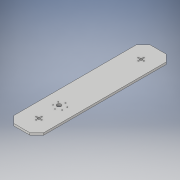
# Autodesk Inventor part: testPart_chassis2
Saved by Autodesk Inventor 2019 (Build 230136000, 136)
## iProperties
Created: 2019-09-17
Part Number: testPart_chassis2
Material: Generic
Document SubType Name: Modeling
Designer: shrey
Density: 1 g/cm^3
Appearance: Default
Author: shrey
Autodesk Inventor part; units mm, degrees
ref_plane "YZ Plane" through (0, 0, 0) normal (1, 0, 0) x (0, 1, 0)
ref_plane "XZ Plane" through (0, 0, 0) normal (0, 1, 0) x (-1, 0, 0)
ref_plane "XY Plane" through (0, 0, 0) normal (0, 0, 1) x (1, 0, 0)
sketch "Sketch1" plane through (0, 0, 0) normal (0, 1, 0) x (-1, 0, 0)
  line L0 (-44.45, -203.2) -> (44.45, -203.2)
  line L1 (44.45, -203.2) -> (44.45, 203.2)
  line L2 (44.45, 203.2) -> (-44.45, 203.2)
  line L3 (-44.45, 203.2) -> (-44.45, -203.2)
  line L4 (-44.45, -203.2) -> (44.45, 203.2) construction
  line L5 (44.45, -203.2) -> (-44.45, 203.2) construction
  line L6 (0, 203.2) -> (0, -203.2) construction
  line L7 (0, 0) -> (44.45, 0) construction
  line L8 (0, -203.2) -> (0, 203.2) construction
  line L9 (0, 152.4) -> (7.112, 152.4) construction
  line L10 (0, -152.4) -> (0, -203.2) construction
  circle A0 centre (0, -152.4) radius 4
  circle A1 centre (0, -152.4) radius 8 construction
  line L11 (0, 152.4) -> (-44.45, 152.4) construction
  line L12 (-44.45, 152.4) -> (-44.45, 88.9)
  line L13 (-44.45, 88.9) -> (0, 88.9) construction
  line L14 (0, 88.9) -> (0, 152.4) construction
  circle A2 centre (0, 88.9) radius 3.556 construction
  circle A3 centre (3.556, 88.9) radius 5.9944
  circle A4 centre (0, 88.9) radius 15.494 construction
  circle A5 centre (0, 104.394) radius 1.5
  circle A6 centre (0, 88.9) radius 15.494 construction
  circle A7 centre (-13.4182, 96.647) radius 1.5
  circle A8 centre (0, 88.9) radius 15.494 construction
  circle A9 centre (-13.4182, 81.153) radius 1.5
  circle A10 centre (0, 88.9) radius 15.494 construction
  circle A11 centre (0, 73.406) radius 1.5
  circle A12 centre (0, 88.9) radius 15.494 construction
  circle A13 centre (13.4182, 81.153) radius 1.5
  circle A14 centre (0, 88.9) radius 15.494 construction
  circle A15 centre (13.4182, 96.647) radius 1.5
  circle A16 centre (0, -144.4) radius 1.85
  circle A17 centre (-8, -152.4) radius 1.85
  circle A18 centre (0, -160.4) radius 1.85
  circle A19 centre (8, -152.4) radius 1.85
  circle A20 centre (0, 152.4) radius 4
  circle A21 centre (0, 152.4) radius 8 construction
  circle A22 centre (0, 160.4) radius 1.85
  circle A23 centre (0, 152.4) radius 8 construction
  circle A24 centre (-8, 152.4) radius 1.85
  circle A25 centre (0, 152.4) radius 8 construction
  circle A26 centre (0, 144.4) radius 1.85
  circle A27 centre (0, 152.4) radius 8 construction
  circle A28 centre (8, 152.4) radius 1.85
  dimension "d17" = 16
  dimension "d26" = 7.112
  dimension "d28" = 30.988
  dimension "d40" = 16
  dimension "d0" = 406.4
  dimension "d1" = 88.9
  dimension "d2" = 152.4
  dimension "d16" = 8
  dimension "d24" = 44.45
  dimension "d25" = 63.5
  dimension "d27" = 11.9888
  dimension "d29" = 3
  dimension "d32" = 360
  dimension "d34" = 3.7
  dimension "d37" = 360
  dimension "d39" = 8
  dimension "d41" = 3.7
  dimension "d44" = 360
  constraints: 30 end point, 17 centre point, 9 coincident, 5 midpoint, 5 vertical alignment, 4 parallel, 4 point on line, 3 horizontal, 3 horizontal alignment, 3 symmetric about line, 2 perpendicular, 1 collinear, 77 other
  measures "d0" distance of L0.end L1.end
  measures "d1" distance of L1.end L2.end
  measures "d2" distance of L7.start point (0, 152.4)
  measures "d16" diameter of A0
  measures "d24" distance of L9.start L11.end
  measures "d25" distance of L11.end L12.end
  measures "d27" diameter of A3
  measures "d29" diameter of A5
  measures "d34" diameter of A16
  measures "d39" diameter of A20
  measures "d41" diameter of A22
extrude "Extrusion2" add sketch "Sketch1" along normal blind 6.35
chamfer "Chamfer2" distance 20.32 angle 45 4 edges at (-44.45, 3.175, -203.2) (-44.45, 3.175, 203.2) (44.45, 3.175, -203.2) (44.45, 3.175, 203.2)
body "Solid2"
